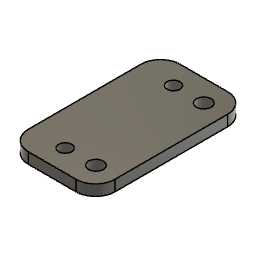
BNO_Mount v3 (Autodesk Fusion 360 design; units mm, degrees)
Autodesk Fusion 360 part; units mm, degrees
sketch "Sketch1" plane through (0, 0, 0) normal (0, 1, 0) x (1, 0, 0)
  line L0 (0, 0) -> (20, 0)
  line L1 (20, 0) -> (20, 35)
  line L2 (20, 35) -> (0, 35)
  line L3 (0, 35) -> (0, 0)
  circle A0 centre (15, 5.1) radius 1.7
  circle A1 centre (15, 30) radius 1.7
  circle A2 centre (8, 5) radius 1.5
  circle A3 centre (8, 30) radius 1.5
  dimension "d1" = 20
  dimension "d2" = 35
  dimension "d3" = 3.4
  dimension "d4" = 3.4
  dimension "d5" = 24.9
  dimension "d6" = 5.1
  dimension "d7" = 5
  dimension "d8" = 5
  dimension "d9" = 3
  dimension "d10" = 3
  dimension "d11" = 25
  dimension "d12" = 7
  dimension "d13" = 7
  dimension "d14" = 5
  constraint horizontal L0
  constraint vertical L1
  constraint horizontal L2
  constraint vertical L3
  constraint coincident L0.start L3.end
  measures "d1" distance of L0.start L0.end
  measures "d2" distance of L0.start L2.end
  measures "d3" diameter of A0
  measures "d4" diameter of A1
  measures "d5" vertical distance of A0.centre A1.centre
  measures "d6" distance of L0 A0.centre
  measures "d7" distance of L1 A1.centre
  measures "d8" distance of L1 A0.centre
  measures "d9" diameter of A2
  measures "d10" diameter of A3
  measures "d11" vertical distance of A2.centre A3.centre
  measures "d12" horizontal distance of A1.centre A3.centre
  measures "d13" horizontal distance of A0.centre A2.centre
  measures "d14" distance of L0 A2.centre
extrude "Extrude1" add sketch "Sketch1" along normal blind 2.5
fillet "Fillet1" radius 4.5 4 edges at (0, 1.25, 0) (20, 1.25, 0) (20, 1.25, -35) (0, 1.25, -35)
